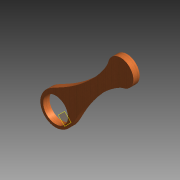
# Autodesk Inventor part: body_11
Saved by Autodesk Inventor 2013 (Build 170138000, 138)
## iProperties
Created: 2013-02-19
Part Number: body_11
Material: Wood (Cherry)
Document SubType Name: Modeling
Designer: Nano
Density: 0.5 g/cm^3
Mass: 10362.4 g
Surface Area: 8680.99 cm^2
Volume: 20724.8 cm^3
Author: Nano
Autodesk Inventor part; units mm, degrees
ref_plane "YZ Plane" through (0, 0, 0) normal (1, 0, 0) x (0, 1, 0)
ref_plane "XZ Plane" through (0, 0, 0) normal (0, 1, 0) x (-1, 0, 0)
ref_plane "XY Plane" through (0, 0, 0) normal (0, 0, 1) x (1, 0, 0)
ref_plane "Work Plane1" through (-34.717, -83.8143, 0) normal (0, 0, 1) x (0.7071068, -0.7071068, 0)
sketch "Sketch1" plane through (-34.717, -83.8143, 0) normal (0, 0, 1) x (0.7071068, -0.7071068, 0)
  circle A0 centre (-118.5314, 0) radius 6.35 projected
  circle A1 centre (-118.5314, 0) radius 149.2286
  arc A2 (48.5793, -75.4462) -> (-285.6421, -75.4462) centre (-118.5314, 0) ccw
  line L0 (-118.5314, 0) -> (-118.5314, 1222.8979) construction
  arc A3 (-244.8846, 1019.4057) -> (7.8218, 1019.4057) centre (-118.5314, 1104.615) ccw
  spline S0 degree 4 poles (7.8218, 1019.4057) (-1.0141, 1006.3032) (-93.9266, 779.7539) (-33.3424, 173.1728) (121.6356, 88.448) (48.5793, -75.4462) knots 0 0 0 0 0 0.357253 1 1 1 1 1
  line L1 (25.7608, 1046.0066) -> (-10.1171, 992.8047) construction
  arc A4 (22.6721, 1027.6714) -> (5.7241, 1002.54) centre (23.3916, 1008.9058) ccw construction
  spline S1 degree 4 poles (-244.8846, 1019.4057) (-236.0486, 1006.3032) (-143.1361, 779.7539) (-203.7203, 173.1728) (-358.6983, 88.448) (-285.6421, -75.4462) knots 0 0 0 0 0 0.357253 1 1 1 1 1
  line L2 (-262.8235, 1046.0066) -> (-226.9456, 992.8047) construction
  arc A5 (-242.7868, 1002.54) -> (-259.7348, 1027.6714) centre (-260.4543, 1008.9058) ccw construction
  arc A6 (-285.6421, -75.4462) -> (48.5793, -75.4462) centre (-118.5314, 0) ccw
  arc A7 (7.8218, 1019.4057) -> (-244.8846, 1019.4057) centre (-118.5314, 1104.615) ccw
  point P0 (-34.717, 83.8143)
  point P1 (-21.2914, 931.7339)
  point P2 (-26.0152, 453.6887)
  point P3 (59.9573, 110.7433)
  point P4 (-215.7713, 931.7339)
  point P5 (-211.0475, 453.6887)
  point P6 (-297.02, 110.7433)
  dimension "d0" = 304.8
  constraints: 10 point on circle, 10 symmetric about line, 7 centre point, 6 end point, 3 midpoint, 2 tangent, 19 other
  measures "d0" diameter of A3
extrude "Extrusion1" add sketch "Sketch1" against normal blind 76.2 contours S0 A2 | A6 S1 A2 S0 | A2 S1 A3 S0 | A2 S1 | A3 A7
body "Solid1"
